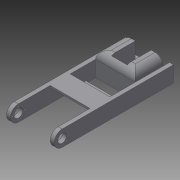
# Autodesk Inventor part: femur
Saved by Autodesk Inventor 2015 (Build 190159000, 159)
## iProperties
Created: 2016-09-30
Part Number: femur
Material: Generic
Document SubType Name: Modeling
Designer: Bardo91
Density: 1 g/cm^3
Appearance: Default
Author: Bardo91
Autodesk Inventor part; units mm, degrees
ref_plane "YZ Plane" through (0, 0, 0) normal (1, 0, 0) x (0, 1, 0)
ref_plane "XZ Plane" through (0, 0, 0) normal (0, 1, 0) x (-1, 0, 0)
ref_plane "XY Plane" through (0, 0, 0) normal (0, 0, 1) x (1, 0, 0)
sketch "Sketch1" plane through (0, 0, 0) normal (0, 0, 1) x (1, 0, 0)
  line L0 (0, 0) -> (-25, 0)
  line L1 (-25, 0) -> (-25, 150)
  line L2 (-25, 150) -> (-30, 150)
  line L3 (-30, 150) -> (-30, 0)
  line L4 (-30, 0) -> (-25, 0)
  line L5 (0, 0) -> (25, 0)
  line L6 (25, 0) -> (25, 150)
  line L7 (25, 150) -> (30, 150)
  line L8 (30, 150) -> (30, 0)
  line L9 (30, 0) -> (25, 0)
  dimension "d0" = 25
  dimension "d1" = 150
  dimension "d2" = 5
  dimension "d3" = 25
  dimension "d4" = 5
  constraints: 20 end point, 6 perpendicular, 5 point on line, 1 horizontal, 1 parallel
  measures "d0" distance of L0.start L0.end
  measures "d1" distance of L0.end L1.end
  measures "d2" distance of L1.end L2.end
  measures "d3" distance of L0.start L5.end
  measures "d4" distance of L6.end L7.end
extrude "Extrusion1" add sketch "Sketch1" along normal blind 20
fillet "Fillet1" radius 10 4 edges at (27.5, 0, 20) (-27.5, 0, 20) (-27.5, 0, 0) (27.5, 0, 0)
sketch "Sketch2" plane through (30, 10, 0) normal (1, 0, 0) x (0, 0, -1)
  arc A0 (-20, 0) -> (0, 0) centre (-10, 0) ccw projected
  line L0 (-10, 0) -> (-20, 0)
  circle A1 centre (-10, 0) radius 5.5
  line L1 (-10, 0) -> (-17.5, 0)
  circle A2 centre (-17.5, 0) radius 0.75
  circle A3 centre (-15.3033, -5.3033) radius 0.75
  circle A4 centre (-10, -7.5) radius 0.75
  circle A5 centre (-4.6967, -5.3033) radius 0.75
  circle A6 centre (-2.5, 0) radius 0.75
  circle A7 centre (-4.6967, 5.3033) radius 0.75
  circle A8 centre (-10, 7.5) radius 0.75
  circle A9 centre (-15.3033, 5.3033) radius 0.75
  point P0 (0, -10)
  dimension "d8" = 11
  dimension "d11" = 7.5
  dimension "d12" = 1.5
  dimension "d15" = 360
  constraints: 9 centre point, 4 end point, 2 coincident, 1 point on circle, 1 point on line, 17 other
  measures "d8" diameter of A1
  measures "d11" distance of L1.start L1.end
  measures "d12" diameter of A2
extrude "Extrusion2" cut sketch "Sketch2" against normal through all
sketch "Sketch3" plane through (30, 10, 0) normal (1, 0, 0) x (0, 0, -1)
  line L0 (0, 0) -> (-20, 0)
  line L1 (-20, 140) -> (-20, 0) projected
  line L2 (-20, 0) -> (-20, 40)
  line L3 (-20, 40) -> (-17.5, 40)
  line L4 (-17.5, 40) -> (-17.5, 65)
  line L5 (-17.5, 65) -> (-20, 65)
  line L6 (-20, 40) -> (-20, 65)
  line L7 (0, 0) -> (0, 60)
  line L8 (0, 60) -> (-2.5, 60)
  line L9 (-2.5, 60) -> (-2.5, 85)
  line L10 (-2.5, 85) -> (0, 85)
  line L11 (0, 85) -> (0, 60)
  line L12 (0, 0) -> (0, 140) projected
  point P0 (0, -10)
  point P1 (-20, 130)
  point P2 (0, 130)
  dimension "d17" = 40
  dimension "d18" = 2.5
  dimension "d19" = 25
  dimension "d20" = 60
  dimension "d21" = 2.5
  dimension "d22" = 25
  constraints: 22 end point, 5 perpendicular, 3 point on line, 2 collinear, 1 horizontal, 1 parallel
  measures "d17" distance of L0.end L2.end
  measures "d18" distance of L2.end L3.end
  measures "d19" distance of L3.end L4.end
  measures "d20" distance of L0.start L7.end
  measures "d21" distance of L7.end L8.end
  measures "d22" distance of L8.end L9.end
extrude "Extrusion3" add sketch "Sketch3" against normal up to surface (60 mm away)
sketch "Sketch9" plane through (0, 0, 0) normal (0, 0, -1) x (-1, 0, 0)
  line L0 (-25, 150) -> (25, 150)
  line L1 (0, 150) -> (-10, 150)
  line L2 (0, 150) -> (10, 150)
  line L3 (-10, 150) -> (-10, 142)
  line L4 (-10, 142) -> (10, 142)
  line L5 (10, 142) -> (10, 150)
  line L6 (10, 142) -> (25, 142)
  line L7 (-10, 142) -> (-25, 142)
  line L8 (-25, 150) -> (-25, 95) projected
  line L9 (25, 150) -> (25, 142)
  line L10 (25, 95) -> (25, 150) projected
  point P0 (0, 0)
  dimension "d49" = 10
  dimension "d50" = 10
  dimension "d51" = 8
  dimension "d52" = 20
  constraints: 18 end point, 3 horizontal, 3 point on line, 2 perpendicular, 1 collinear, 1 midpoint
  measures "d49" distance of L1.start L1.end
  measures "d50" distance of L1.start L2.end
  measures "d51" distance of L1.end L3.end
  measures "d52" distance of L3.end L4.end
extrude "Extrusion9" add sketch "Sketch9" against normal blind 7
sketch "Sketch10" plane through (0, 0, 0) normal (0, 0, -1) x (-1, 0, 0)
  line L0 (25, 142) -> (-25, 142) projected
  line L1 (0, 142) -> (-10, 142)
  line L2 (-10, 142) -> (-10, 112)
  line L3 (-10, 112) -> (10, 112)
  line L4 (10, 112) -> (10, 142)
  line L5 (-10, 142) -> (-25, 142)
  line L6 (-25, 142) -> (-25, 107)
  line L7 (-25, 142) -> (-25, 95) projected
  line L8 (-25, 107) -> (25, 107)
  line L9 (25, 75) -> (25, 150) projected
  line L10 (10, 142) -> (25, 142)
  line L11 (25, 142) -> (25, 107)
  point P0 (0, 0)
  dimension "d55" = 10
  dimension "d56" = 30
  dimension "d57" = 20
  dimension "d58" = 35
  constraints: 18 end point, 4 perpendicular, 4 point on line, 3 collinear, 1 midpoint
  measures "d55" distance of L1.start L1.end
  measures "d56" distance of L1.end L2.end
  measures "d57" distance of L2.end L3.end
  measures "d58" distance of L0.end L6.end
extrude "Extrusion10" add sketch "Sketch10" against normal blind 30 contours L9 L8 L6 L0 L2 L3 L4
fillet "Fillet2" radius 10 3 edges at (-25, 124.5, 30) (25, 124.5, 30) (0, 107, 30)
sketch "Sketch11" plane through (-30, 150, 0) normal (0, 1, 0) x (1, 0, 0)
  line L0 (30, 0) -> (30, -2.5)
  line L1 (30, -2.5) -> (25, -2.5)
  line L2 (55, -2.5) -> (5, -2.5) projected
  line L3 (25, -2.5) -> (35, -2.5)
  circle A0 centre (25, -2.5) radius 2.75
  circle A1 centre (35, -2.5) radius 2.75
  dimension "d62" = 2.5
  dimension "d63" = 5
  dimension "d64" = 10
  dimension "d65" = 5.5
  dimension "d66" = 5.5
  constraints: 6 end point, 2 centre point, 2 coincident, 2 point on line, 1 vertical
  measures "d62" distance of L0.start L0.end
  measures "d63" distance of L0.end L1.end
  measures "d64" distance of L1.end L3.end
  measures "d65" diameter of A0
  measures "d66" diameter of A1
extrude "Extrusion11" cut sketch "Sketch11" against normal blind 30
equation "\"d9\" = d8"
body "Solid1"
